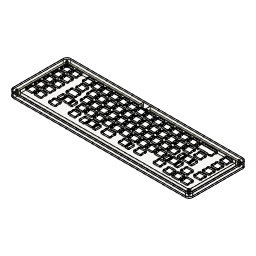
FrogdorCase (Autodesk Fusion 360 design; units mm, degrees)
Autodesk Fusion 360 part; units mm, degrees
(part 1 of 5)
sketch "plate" plane through (0, 0, 0) normal (0, 0, 1) x (1, 0, 0)
  line L0 (288.37, 77.8715) -> (287.569, 77.8715)
  line L1 (326.182, 65.8717) -> (326.981, 65.8717)
  line L2 (17.4198, 49.9223) -> (16.6192, 49.9223)
  line L3 (350.282, 78.8719) -> (350.282, 77.8715)
  line L4 (312.182, 68.9723) -> (311.381, 68.9723)
  line L5 (326.981, 65.8717) -> (326.981, 68.9723)
  line L6 (365.083, 65.8717) -> (365.083, 68.9723)
  line L7 (312.182, 77.8715) -> (311.381, 77.8715)
  line L8 (312.182, 64.8727) -> (326.182, 64.8727)
  line L9 (311.381, 74.7723) -> (312.182, 74.7723)
  line L10 (287.569, 77.8715) -> (287.569, 74.7723)
  line L11 (287.569, 74.7723) -> (288.37, 74.7723)
  line L12 (364.282, 77.8715) -> (364.282, 78.8719)
  line L13 (326.182, 74.7723) -> (326.981, 74.7723)
  line L14 (288.37, 68.9723) -> (287.569, 68.9723)
  line L15 (288.37, 74.7723) -> (288.37, 68.9723)
  line L16 (288.37, 65.8717) -> (288.37, 64.8727)
  line L17 (16.6192, 58.8215) -> (16.6192, 59.8219)
  line L18 (326.981, 74.7723) -> (326.981, 77.8715)
  line L19 (350.282, 64.8727) -> (364.282, 64.8727)
  line L20 (365.083, 68.9723) -> (364.282, 68.9723)
  line L21 (287.569, 68.9723) -> (287.569, 65.8717)
  line L22 (349.481, 65.8717) -> (350.282, 65.8717)
  line L23 (311.381, 77.8715) -> (311.381, 74.7723)
  line L24 (364.282, 74.7723) -> (365.083, 74.7723)
  line L25 (350.282, 77.8715) -> (349.481, 77.8715)
  line L26 (364.282, 68.9723) -> (364.282, 74.7723)
  line L27 (16.6192, 59.8219) -> (2.6196, 59.8219)
  line L28 (365.083, 77.8715) -> (364.282, 77.8715)
  line L29 (326.182, 77.8715) -> (326.182, 78.8719)
  line L30 (16.6192, 55.7223) -> (17.4198, 55.7223)
  line L31 (326.981, 68.9723) -> (326.182, 68.9723)
  line L32 (288.37, 64.8727) -> (302.369, 64.8727)
  line L33 (302.369, 65.8717) -> (303.17, 65.8717)
  line L34 (326.182, 64.8727) -> (326.182, 65.8717)
  line L35 (303.17, 65.8717) -> (303.17, 68.9723)
  line L36 (365.083, 74.7723) -> (365.083, 77.8715)
  line L37 (303.17, 68.9723) -> (302.369, 68.9723)
  line L38 (326.981, 77.8715) -> (326.182, 77.8715)
  line L39 (349.481, 74.7723) -> (350.282, 74.7723)
  line L40 (312.182, 65.8717) -> (312.182, 64.8727)
  line L41 (326.182, 68.9723) -> (326.182, 74.7723)
  line L42 (350.282, 68.9723) -> (349.481, 68.9723)
  line L43 (231.22, 74.7723) -> (231.22, 68.9723)
  line L44 (249.469, 65.8717) -> (250.27, 65.8717)
  line L45 (283.319, 68.9723) -> (283.319, 74.7723)
  line L46 (264.269, 77.8715) -> (264.269, 78.8719)
  line L47 (268.519, 74.7723) -> (269.32, 74.7723)
  line L48 (230.419, 77.8715) -> (230.419, 74.7723)
  line L49 (265.07, 77.8715) -> (264.269, 77.8715)
  line L50 (265.07, 65.8717) -> (265.07, 68.9723)
  line L51 (230.419, 68.9723) -> (230.419, 65.8717)
  line L52 (231.22, 78.8719) -> (231.22, 77.8715)
  line L53 (264.269, 65.8717) -> (265.07, 65.8717)
  line L54 (250.27, 78.8719) -> (250.27, 77.8715)
  line L55 (302.369, 64.8727) -> (302.369, 65.8717)
  line L56 (231.22, 77.8715) -> (230.419, 77.8715)
  line L57 (230.419, 74.7723) -> (231.22, 74.7723)
  line L58 (249.469, 74.7723) -> (250.27, 74.7723)
  line L59 (268.519, 68.9723) -> (268.519, 65.8717)
  line L60 (268.519, 65.8717) -> (269.32, 65.8717)
  line L61 (269.32, 65.8717) -> (269.32, 64.8727)
  line L62 (287.569, 65.8717) -> (288.37, 65.8717)
  line L63 (302.369, 78.8719) -> (288.37, 78.8719)
  line L64 (326.182, 78.8719) -> (312.182, 78.8719)
  line L65 (283.319, 64.8727) -> (283.319, 65.8717)
  line L66 (302.369, 77.8715) -> (302.369, 78.8719)
  line L67 (349.481, 68.9723) -> (349.481, 65.8717)
  line L68 (246.02, 65.8717) -> (246.02, 68.9723)
  line L69 (269.32, 74.7723) -> (269.32, 68.9723)
  line L70 (245.219, 65.8717) -> (246.02, 65.8717)
  line L71 (245.219, 68.9723) -> (245.219, 74.7723)
  line L72 (350.282, 65.8717) -> (350.282, 64.8727)
  line L73 (284.12, 65.8717) -> (284.12, 68.9723)
  line L74 (212.17, 78.8719) -> (212.17, 77.8715)
  line L75 (245.219, 78.8719) -> (231.22, 78.8719)
  line L76 (250.27, 77.8715) -> (249.469, 77.8715)
  line L77 (245.219, 77.8715) -> (245.219, 78.8719)
  line L78 (283.319, 65.8717) -> (284.12, 65.8717)
  line L79 (283.319, 78.8719) -> (269.32, 78.8719)
  line L80 (265.07, 74.7723) -> (265.07, 77.8715)
  line L81 (250.27, 65.8717) -> (250.27, 64.8727)
  line L82 (231.22, 65.8717) -> (231.22, 64.8727)
  line L83 (283.319, 77.8715) -> (283.319, 78.8719)
  line L84 (264.269, 74.7723) -> (265.07, 74.7723)
  line L85 (246.02, 74.7723) -> (246.02, 77.8715)
  line L86 (268.519, 77.8715) -> (268.519, 74.7723)
  line L87 (249.469, 77.8715) -> (249.469, 74.7723)
  line L88 (302.369, 74.7723) -> (303.17, 74.7723)
  line L89 (230.419, 65.8717) -> (231.22, 65.8717)
  line L90 (231.22, 64.8727) -> (245.219, 64.8727)
  line L91 (246.02, 68.9723) -> (245.219, 68.9723)
  line L92 (246.02, 77.8715) -> (245.219, 77.8715)
  line L93 (269.32, 64.8727) -> (283.319, 64.8727)
  line L94 (303.17, 74.7723) -> (303.17, 77.8715)
  line L95 (264.269, 68.9723) -> (264.269, 74.7723)
  line L96 (245.219, 64.8727) -> (245.219, 65.8717)
  line L97 (249.469, 68.9723) -> (249.469, 65.8717)
  line L98 (250.27, 64.8727) -> (264.269, 64.8727)
  line L99 (231.22, 68.9723) -> (230.419, 68.9723)
  line L100 (265.07, 68.9723) -> (264.269, 68.9723)
  line L101 (245.219, 74.7723) -> (246.02, 74.7723)
  line L102 (264.269, 78.8719) -> (250.27, 78.8719)
  line L103 (284.12, 68.9723) -> (283.319, 68.9723)
  line L104 (264.269, 64.8727) -> (264.269, 65.8717)
  line L105 (269.32, 77.8715) -> (268.519, 77.8715)
  line L106 (283.319, 74.7723) -> (284.12, 74.7723)
  line L107 (250.27, 74.7723) -> (250.27, 68.9723)
  line L108 (226.169, 78.8719) -> (212.17, 78.8719)
  line L109 (193.12, 68.9723) -> (192.319, 68.9723)
  line L110 (193.12, 78.8719) -> (193.12, 77.8715)
  line L111 (226.97, 65.8717) -> (226.97, 68.9723)
  line L112 (188.069, 64.8727) -> (188.069, 65.8717)
  line L113 (250.27, 68.9723) -> (249.469, 68.9723)
  line L114 (193.12, 65.8717) -> (193.12, 64.8727)
  line L115 (174.07, 74.7723) -> (174.07, 68.9723)
  line L116 (269.32, 68.9723) -> (268.519, 68.9723)
  line L117 (303.17, 77.8715) -> (302.369, 77.8715)
  line L118 (192.319, 77.8715) -> (192.319, 74.7723)
  line L119 (192.319, 65.8717) -> (193.12, 65.8717)
  line L120 (188.069, 65.8717) -> (188.87, 65.8717)
  line L121 (212.17, 68.9723) -> (211.369, 68.9723)
  line L122 (226.97, 74.7723) -> (226.97, 77.8715)
  line L123 (155.02, 78.8719) -> (155.02, 77.8715)
  line L124 (226.97, 68.9723) -> (226.169, 68.9723)
  line L125 (226.169, 74.7723) -> (226.97, 74.7723)
  line L126 (207.119, 68.9723) -> (207.119, 74.7723)
  line L127 (284.12, 77.8715) -> (283.319, 77.8715)
  line L128 (226.169, 77.8715) -> (226.169, 78.8719)
  line L129 (226.169, 64.8727) -> (226.169, 65.8717)
  line L130 (188.87, 65.8717) -> (188.87, 68.9723)
  line L131 (192.319, 74.7723) -> (193.12, 74.7723)
  line L132 (207.119, 74.7723) -> (207.92, 74.7723)
  line L133 (154.219, 77.8715) -> (154.219, 74.7723)
  line L134 (193.12, 77.8715) -> (192.319, 77.8715)
  line L135 (188.069, 74.7723) -> (188.87, 74.7723)
  line L136 (192.319, 68.9723) -> (192.319, 65.8717)
  line L137 (188.87, 74.7723) -> (188.87, 77.8715)
  line L138 (174.07, 68.9723) -> (173.269, 68.9723)
  line L139 (154.219, 74.7723) -> (155.02, 74.7723)
  line L140 (193.12, 74.7723) -> (193.12, 68.9723)
  line L141 (155.02, 74.7723) -> (155.02, 68.9723)
  line L142 (188.069, 77.8715) -> (188.069, 78.8719)
  line L143 (211.369, 77.8715) -> (211.369, 74.7723)
  line L144 (212.17, 74.7723) -> (212.17, 68.9723)
  line L145 (207.92, 65.8717) -> (207.92, 68.9723)
  line L146 (207.92, 68.9723) -> (207.119, 68.9723)
  line L147 (269.32, 78.8719) -> (269.32, 77.8715)
  line L148 (284.12, 74.7723) -> (284.12, 77.8715)
  line L149 (226.97, 77.8715) -> (226.169, 77.8715)
  line L150 (188.069, 68.9723) -> (188.069, 74.7723)
  line L151 (193.12, 64.8727) -> (207.119, 64.8727)
  line L152 (188.069, 78.8719) -> (174.07, 78.8719)
  line L153 (155.02, 77.8715) -> (154.219, 77.8715)
  line L154 (207.119, 77.8715) -> (207.119, 78.8719)
  line L155 (207.92, 74.7723) -> (207.92, 77.8715)
  line L156 (174.07, 64.8727) -> (188.069, 64.8727)
  line L157 (211.369, 74.7723) -> (212.17, 74.7723)
  line L158 (211.369, 65.8717) -> (212.17, 65.8717)
  line L159 (173.269, 65.8717) -> (174.07, 65.8717)
  line L160 (188.87, 77.8715) -> (188.069, 77.8715)
  line L161 (188.87, 68.9723) -> (188.069, 68.9723)
  line L162 (173.269, 74.7723) -> (174.07, 74.7723)
  line L163 (207.119, 65.8717) -> (207.92, 65.8717)
  line L164 (173.269, 68.9723) -> (173.269, 65.8717)
  line L165 (174.07, 65.8717) -> (174.07, 64.8727)
  line L166 (94.6877, 11.8222) -> (94.6877, 8.7216)
  line L167 (16.6192, 8.7216) -> (17.4198, 8.7216)
  line L168 (326.47, 23.0105) -> (326.47, 22.01)
  line L169 (325.669, 31.9098) -> (326.47, 31.9098)
  line L170 (36.4698, 17.6237) -> (36.4698, 20.7216)
  line L171 (238.362, 17.6237) -> (238.362, 11.8222)
  line L172 (16.6192, 21.722) -> (2.6196, 21.722)
  line L173 (109.488, 20.7216) -> (109.488, 21.722)
  line L174 (51.8252, 20.7216) -> (51.8252, 17.6237)
  line L175 (340.469, 36.0094) -> (326.47, 36.0094)
  line L176 (66.6253, 21.722) -> (52.626, 21.722)
  line L177 (66.6253, 20.7216) -> (66.6253, 21.722)
  line L178 (109.488, 17.6237) -> (110.287, 17.6237)
  line L179 (67.4261, 17.6237) -> (67.4261, 20.7216)
  line L180 (340.469, 22.01) -> (340.469, 23.0105)
  line L181 (341.27, 26.1097) -> (340.469, 26.1097)
  line L182 (17.4198, 20.7216) -> (16.6192, 20.7216)
  line L183 (325.669, 35.0104) -> (325.669, 31.9098)
  line L184 (325.669, 23.0105) -> (326.47, 23.0105)
  line L185 (35.669, 7.7225) -> (35.669, 8.7216)
  line L186 (293.132, 39.7715) -> (292.331, 39.7715)
  line L187 (17.4198, 17.6237) -> (17.4198, 20.7216)
  line L188 (67.4261, 8.7216) -> (67.4261, 11.8222)
  line L189 (110.287, 20.7216) -> (109.488, 20.7216)
  line L190 (326.47, 35.0104) -> (325.669, 35.0104)
  line L191 (341.27, 31.9098) -> (341.27, 35.0104)
  line L192 (21.6697, 7.7225) -> (35.669, 7.7225)
  line L193 (340.469, 26.1097) -> (340.469, 31.9098)
  line L194 (341.27, 23.0105) -> (341.27, 26.1097)
  line L195 (95.4871, 7.7225) -> (109.488, 7.7225)
  line L196 (35.669, 8.7216) -> (36.4698, 8.7216)
  line L197 (1.819, 11.8222) -> (1.819, 8.7216)
  line L198 (340.469, 35.0104) -> (340.469, 36.0094)
  line L199 (237.563, 11.8222) -> (237.563, 8.7216)
  line L200 (16.6192, 11.8222) -> (16.6192, 17.6237)
  line L201 (16.6192, 17.6237) -> (17.4198, 17.6237)
  line L202 (16.6192, 20.7216) -> (16.6192, 21.722)
  line L203 (1.819, 8.7216) -> (2.6197, 8.7216)
  line L204 (293.132, 36.6723) -> (293.132, 36.0715)
  line L205 (326.47, 22.01) -> (340.469, 22.01)
  line L206 (2.6197, 8.7216) -> (2.6197, 7.7225)
  line L207 (66.6253, 7.7225) -> (66.6253, 8.7216)
  line L208 (1.819, 17.6237) -> (2.6197, 17.6237)
  line L209 (52.626, 20.7216) -> (51.8252, 20.7216)
  line L210 (110.287, 8.7216) -> (110.287, 11.8222)
  line L211 (1.819, 20.7216) -> (1.819, 17.6237)
  line L212 (36.4698, 8.7216) -> (36.4698, 11.8222)
  line L213 (292.331, 36.6723) -> (293.132, 36.6723)
  line L214 (35.669, 17.6237) -> (36.4698, 17.6237)
  line L215 (326.47, 36.0094) -> (326.47, 35.0104)
  line L216 (17.4198, 8.7216) -> (17.4198, 11.8222)
  line L217 (36.4698, 11.8222) -> (35.669, 11.8222)
  line L218 (17.4198, 11.8222) -> (16.6192, 11.8222)
  line L219 (340.469, 31.9098) -> (341.27, 31.9098)
  line L220 (35.669, 11.8222) -> (35.669, 17.6237)
  line L221 (36.4698, 20.7216) -> (35.669, 20.7216)
  line L222 (341.27, 35.0104) -> (340.469, 35.0104)
  line L223 (21.6697, 8.7216) -> (21.6697, 7.7225)
  line L224 (340.469, 23.0105) -> (341.27, 23.0105)
  line L225 (325.669, 26.1097) -> (325.669, 23.0105)
  line L226 (35.669, 20.7216) -> (35.669, 21.722)
  line L227 (2.6197, 20.7216) -> (1.819, 20.7216)
  line L228 (2.6197, 17.6237) -> (2.6197, 11.8222)
  line L229 (293.132, 40.7719) -> (293.132, 39.7715)
  line L230 (35.669, 21.722) -> (21.6697, 21.722)
  line L231 (284.032, 36.0715) -> (284.032, 33.2727)
  line L232 (292.331, 39.7715) -> (292.331, 36.6723)
  line L233 (291.607, 36.0715) -> (291.607, 38.3016)
  line L234 (326.47, 31.9098) -> (326.47, 26.1097)
  line L235 (326.47, 26.1097) -> (325.669, 26.1097)
  line L236 (2.6197, 7.7225) -> (16.6192, 7.7225)
  line L237 (16.6192, 7.7225) -> (16.6192, 8.7216)
  line L238 (61.3502, 39.7715) -> (61.3502, 36.6737)
  line L239 (291.607, 27.0027) -> (291.607, 31.4716)
  line L240 (307.132, 27.7716) -> (307.931, 27.7716)
  line L241 (307.132, 26.7725) -> (307.132, 27.7716)
  line L242 (315.407, 39.3016) -> (315.248, 39.3016)
  line L243 (307.132, 40.7719) -> (293.132, 40.7719)
  line L244 (62.151, 39.7715) -> (61.3502, 39.7715)
  line L245 (60.6256, 36.0715) -> (60.6256, 39.3016)
  line L246 (61.3502, 36.6737) -> (62.151, 36.6737)
  line L247 (307.132, 39.7715) -> (307.132, 40.7719)
  line L248 (2.6197, 11.8222) -> (1.819, 11.8222)
  line L249 (2.6197, 21.722) -> (2.6197, 20.7216)
  line L250 (293.132, 26.7725) -> (307.132, 26.7725)
  line L251 (62.151, 36.6737) -> (62.151, 36.0715)
  line L252 (61.3502, 30.8722) -> (61.3502, 27.7716)
  line L253 (307.931, 30.8722) -> (307.132, 30.8722)
  line L254 (62.151, 40.7719) -> (62.151, 39.7715)
  line L255 (61.3502, 27.7716) -> (62.151, 27.7716)
  line L256 (60.6225, 27.0027) -> (60.6256, 27.0027)
  line L257 (307.931, 39.7715) -> (307.132, 39.7715)
  line L258 (307.132, 36.6723) -> (307.931, 36.6723)
  line L259 (62.151, 31.4716) -> (62.151, 30.8722)
  line L260 (307.931, 36.6723) -> (307.931, 39.7715)
  line L261 (60.6256, 39.3016) -> (53.8759, 39.3016)
  line L262 (60.6256, 27.0027) -> (60.6256, 31.4716)
  line L263 (316.231, 33.2727) -> (316.231, 36.0715)
  line L264 (62.151, 30.8722) -> (61.3502, 30.8722)
  line L265 (307.132, 30.8722) -> (307.132, 31.4716)
  line L266 (292.331, 27.7716) -> (293.132, 27.7716)
  line L267 (292.331, 30.8722) -> (292.331, 27.7716)
  line L268 (293.132, 27.7716) -> (293.132, 26.7725)
  line L269 (307.931, 27.7716) -> (307.931, 30.8722)
  line L270 (293.132, 31.4716) -> (293.132, 30.8722)
  line L271 (293.132, 30.8722) -> (292.331, 30.8722)
  line L272 (364.282, 36.6737) -> (365.083, 36.6737)
  line L273 (62.151, 27.7716) -> (62.151, 26.7725)
  line L274 (350.282, 39.7715) -> (349.481, 39.7715)
  line L275 (76.1503, 36.6737) -> (76.9511, 36.6737)
  line L276 (76.1503, 40.7719) -> (62.151, 40.7719)
  line L277 (350.282, 26.7725) -> (364.282, 26.7725)
  line L278 (264.557, 30.8722) -> (263.756, 30.8722)
  line L279 (350.282, 36.6737) -> (350.282, 30.8722)
  line L280 (349.481, 30.8722) -> (349.481, 27.7716)
  line L281 (278.557, 27.7716) -> (279.356, 27.7716)
  line L282 (77.676, 31.4716) -> (77.676, 27.0027)
  line L283 (350.282, 30.8722) -> (349.481, 30.8722)
  line L284 (76.9511, 39.7715) -> (76.1503, 39.7715)
  line L285 (76.9511, 36.6737) -> (76.9511, 39.7715)
  line L286 (263.756, 27.7716) -> (264.557, 27.7716)
  line L287 (76.9511, 27.7716) -> (76.9511, 30.8722)
  line L288 (349.481, 39.7715) -> (349.481, 36.6737)
  line L289 (364.282, 40.7719) -> (350.282, 40.7719)
  line L290 (264.557, 27.7716) -> (264.557, 26.7725)
  line L291 (349.481, 27.7716) -> (350.282, 27.7716)
  line L292 (76.1503, 27.7716) -> (76.9511, 27.7716)
  line L293 (365.083, 39.7715) -> (364.282, 39.7715)
  line L294 (307.132, 36.0715) -> (307.132, 36.6723)
  line L295 (263.756, 39.7715) -> (263.756, 36.6737)
  line L296 (365.083, 30.8722) -> (364.282, 30.8722)
  line L297 (264.557, 40.7719) -> (264.557, 39.7715)
  line L298 (62.151, 26.7725) -> (76.1503, 26.7725)
  line L299 (263.756, 30.8722) -> (263.756, 27.7716)
  line L300 (279.356, 27.7716) -> (279.356, 30.8722)
  line L301 (364.282, 26.7725) -> (364.282, 27.7716)
  line L302 (279.356, 30.8722) -> (278.557, 30.8722)
  line L303 (264.557, 26.7725) -> (278.557, 26.7725)
  line L304 (77.676, 38.3016) -> (77.676, 36.0715)
  line L305 (76.9511, 30.8722) -> (76.1503, 30.8722)
  line L306 (76.1503, 36.0715) -> (76.1503, 36.6737)
  line L307 (263.756, 36.6737) -> (264.557, 36.6737)
  line L308 (264.557, 36.6737) -> (264.557, 30.8722)
  line L309 (76.1503, 26.7725) -> (76.1503, 27.7716)
  line L310 (350.282, 27.7716) -> (350.282, 26.7725)
  line L311 (278.557, 26.7725) -> (278.557, 27.7716)
  line L312 (76.1503, 30.8722) -> (76.1503, 31.4716)
  line L313 (278.557, 36.6737) -> (279.356, 36.6737)
  line L314 (76.1503, 39.7715) -> (76.1503, 40.7719)
  line L315 (264.557, 39.7715) -> (263.756, 39.7715)
  line L316 (350.282, 40.7719) -> (350.282, 39.7715)
  line L317 (364.282, 30.8722) -> (364.282, 36.6737)
  line L318 (349.481, 36.6737) -> (350.282, 36.6737)
  line L319 (365.083, 36.6737) -> (365.083, 39.7715)
  line L320 (365.083, 27.7716) -> (365.083, 30.8722)
  line L321 (278.557, 30.8722) -> (278.557, 36.6737)
  line L322 (278.557, 40.7719) -> (264.557, 40.7719)
  line L323 (126.157, 39.7715) -> (126.157, 40.7719)
  line L324 (260.306, 36.6737) -> (260.306, 39.7715)
  line L325 (364.282, 39.7715) -> (364.282, 40.7719)
  line L326 (240.457, 30.8722) -> (240.457, 36.6737)
  line L327 (245.507, 26.7725) -> (259.507, 26.7725)
  line L328 (93.1072, 30.8722) -> (92.3064, 30.8722)
  line L329 (279.356, 36.6737) -> (279.356, 39.7715)
  line L330 (111.356, 36.6737) -> (112.157, 36.6737)
  line L331 (126.157, 27.7716) -> (126.956, 27.7716)
  line L332 (225.656, 27.7716) -> (226.457, 27.7716)
  line L333 (206.606, 36.6737) -> (207.407, 36.6737)
  line L334 (240.457, 36.6737) -> (241.256, 36.6737)
  line L335 (260.306, 30.8722) -> (259.507, 30.8722)
  line L336 (244.706, 27.7716) -> (245.507, 27.7716)
  line L337 (126.956, 36.6737) -> (126.956, 39.7715)
  line L338 (92.3064, 39.7715) -> (92.3064, 36.6737)
  line L339 (130.406, 36.6737) -> (131.207, 36.6737)
  line L340 (207.407, 40.7719) -> (207.407, 39.7715)
  line L341 (93.1072, 40.7719) -> (93.1072, 39.7715)
  line L342 (225.656, 39.7715) -> (225.656, 36.6737)
  line L343 (259.507, 39.7715) -> (259.507, 40.7719)
  line L344 (240.457, 40.7719) -> (226.457, 40.7719)
  line L345 (226.457, 39.7715) -> (225.656, 39.7715)
  line L346 (225.656, 36.6737) -> (226.457, 36.6737)
  line L347 (206.606, 39.7715) -> (206.606, 36.6737)
  line L348 (226.457, 36.6737) -> (226.457, 30.8722)
  line L349 (240.457, 27.7716) -> (241.256, 27.7716)
  line L350 (244.706, 30.8722) -> (244.706, 27.7716)
  line L351 (226.457, 40.7719) -> (226.457, 39.7715)
  line L352 (260.306, 27.7716) -> (260.306, 30.8722)
  line L353 (241.256, 27.7716) -> (241.256, 30.8722)
  line L354 (241.256, 39.7715) -> (240.457, 39.7715)
  line L355 (259.507, 27.7716) -> (260.306, 27.7716)
  line L356 (244.706, 39.7715) -> (244.706, 36.6737)
  line L357 (206.606, 30.8722) -> (206.606, 27.7716)
  line L358 (245.507, 27.7716) -> (245.507, 26.7725)
  line L359 (93.1072, 36.6737) -> (93.1072, 30.8722)
  line L360 (226.457, 27.7716) -> (226.457, 26.7725)
  line L361 (245.507, 40.7719) -> (245.507, 39.7715)
  line L362 (259.507, 26.7725) -> (259.507, 27.7716)
  line L363 (207.407, 30.8722) -> (206.606, 30.8722)
  line L364 (245.507, 30.8722) -> (244.706, 30.8722)
  line L365 (226.457, 26.7725) -> (240.457, 26.7725)
  line L366 (241.256, 36.6737) -> (241.256, 39.7715)
  line L367 (240.457, 26.7725) -> (240.457, 27.7716)
  line L368 (112.157, 39.7715) -> (111.356, 39.7715)
  line L369 (364.282, 27.7716) -> (365.083, 27.7716)
  line L370 (259.507, 36.6737) -> (260.306, 36.6737)
  line L371 (207.407, 39.7715) -> (206.606, 39.7715)
  line L372 (260.306, 39.7715) -> (259.507, 39.7715)
  line L373 (259.507, 30.8722) -> (259.507, 36.6737)
  line L374 (245.507, 36.6737) -> (245.507, 30.8722)
  line L375 (207.407, 36.6737) -> (207.407, 30.8722)
  line L376 (279.356, 39.7715) -> (278.557, 39.7715)
  line L377 (259.507, 40.7719) -> (245.507, 40.7719)
  line L378 (278.557, 39.7715) -> (278.557, 40.7719)
  line L379 (241.256, 30.8722) -> (240.457, 30.8722)
  line L380 (245.507, 39.7715) -> (244.706, 39.7715)
  line L381 (244.706, 36.6737) -> (245.507, 36.6737)
  line L382 (240.457, 39.7715) -> (240.457, 40.7719)
  line L383 (226.457, 30.8722) -> (225.656, 30.8722)
  line L384 (225.656, 30.8722) -> (225.656, 27.7716)
  line L385 (126.157, 36.6737) -> (126.956, 36.6737)
  line L386 (93.1072, 27.7716) -> (93.1072, 26.7725)
  line L387 (21.6697, 40.7719) -> (21.6697, 39.7715)
  line L388 (131.207, 27.7716) -> (131.207, 26.7725)
  line L389 (112.157, 27.7716) -> (112.157, 26.7725)
  line L390 (92.3064, 30.8722) -> (92.3064, 27.7716)
  line L391 (145.207, 27.7716) -> (146.006, 27.7716)
  line L392 (130.406, 30.8722) -> (130.406, 27.7716)
  line L393 (107.906, 27.7716) -> (107.906, 30.8722)
  line L394 (131.207, 40.7719) -> (131.207, 39.7715)
  line L395 (145.207, 26.7725) -> (145.207, 27.7716)
  line L396 (126.956, 30.8722) -> (126.157, 30.8722)
  line L397 (126.956, 27.7716) -> (126.956, 30.8722)
  line L398 (146.006, 30.8722) -> (145.207, 30.8722)
  line L399 (112.157, 40.7719) -> (112.157, 39.7715)
  line L400 (164.257, 39.7715) -> (164.257, 40.7719)
  line L401 (131.207, 26.7725) -> (145.207, 26.7725)
  line L402 (131.207, 30.8722) -> (130.406, 30.8722)
  line L403 (107.107, 36.6737) -> (107.906, 36.6737)
  line L404 (93.1072, 39.7715) -> (92.3064, 39.7715)
  line L405 (111.356, 27.7716) -> (112.157, 27.7716)
  line L406 (145.207, 40.7719) -> (131.207, 40.7719)
  line L407 (107.107, 27.7716) -> (107.906, 27.7716)
  line L408 (112.157, 26.7725) -> (126.157, 26.7725)
  line L409 (146.006, 27.7716) -> (146.006, 30.8722)
  line L410 (92.3064, 27.7716) -> (93.1072, 27.7716)
  line L411 (107.906, 36.6737) -> (107.906, 39.7715)
  line L412 (131.207, 39.7715) -> (130.406, 39.7715)
  line L413 (165.056, 39.7715) -> (164.257, 39.7715)
  line L414 (107.107, 30.8722) -> (107.107, 36.6737)
  line L415 (107.107, 26.7725) -> (107.107, 27.7716)
  line L416 (145.207, 39.7715) -> (145.207, 40.7719)
  line L417 (146.006, 36.6737) -> (146.006, 39.7715)
  line L418 (130.406, 39.7715) -> (130.406, 36.6737)
  line L419 (107.906, 39.7715) -> (107.107, 39.7715)
  line L420 (2.6197, 27.7716) -> (2.6197, 26.7725)
  line L421 (305.037, 55.7223) -> (305.037, 55.1215)
  line L422 (16.6192, 30.8722) -> (16.6192, 36.6737)
  line L423 (16.6192, 27.7716) -> (17.4198, 27.7716)
  line L424 (17.4198, 36.6737) -> (17.4198, 39.7715)
  line L425 (20.869, 27.7716) -> (21.6697, 27.7716)
  line L426 (36.4698, 30.8722) -> (35.669, 30.8722)
  line L427 (304.238, 55.7223) -> (305.037, 55.7223)
  line L428 (126.157, 26.7725) -> (126.157, 27.7716)
  line L429 (20.869, 39.7715) -> (20.869, 36.6737)
  line L430 (35.669, 27.7716) -> (36.4698, 27.7716)
  line L431 (130.406, 27.7716) -> (131.207, 27.7716)
  line L432 (21.6697, 26.7725) -> (35.669, 26.7725)
  line L433 (17.4198, 30.8722) -> (16.6192, 30.8722)
  line L434 (107.107, 39.7715) -> (107.107, 40.7719)
  line L435 (305.037, 59.8219) -> (305.037, 58.8215)
  line L436 (107.906, 30.8722) -> (107.107, 30.8722)
  line L437 (2.6197, 36.6737) -> (2.6197, 30.8722)
  line L438 (2.6197, 30.8722) -> (1.819, 30.8722)
  line L439 (305.037, 50.5217) -> (305.037, 49.9223)
  line L440 (305.037, 49.9223) -> (304.238, 49.9223)
  line L441 (16.6192, 39.7715) -> (16.6192, 40.7719)
  line L442 (305.037, 58.8215) -> (304.238, 58.8215)
  line L443 (35.669, 39.7715) -> (35.669, 40.7719)
  line L444 (112.157, 30.8722) -> (111.356, 30.8722)
  line L445 (1.819, 27.7716) -> (2.6197, 27.7716)
  line L446 (2.6197, 26.7725) -> (16.6192, 26.7725)
  line L447 (2.6197, 39.7715) -> (1.819, 39.7715)
  line L448 (21.6697, 36.6737) -> (21.6697, 30.8722)
  line L449 (145.207, 30.8722) -> (145.207, 36.6737)
  line L450 (36.4698, 39.7715) -> (35.669, 39.7715)
  line L451 (126.157, 40.7719) -> (112.157, 40.7719)
  line L452 (164.257, 40.7719) -> (150.257, 40.7719)
  line L453 (1.819, 36.6737) -> (2.6197, 36.6737)
  line L454 (111.356, 39.7715) -> (111.356, 36.6737)
  line L455 (17.4198, 27.7716) -> (17.4198, 30.8722)
  line L456 (303.513, 55.1215) -> (303.513, 57.3516)
  line L457 (92.3064, 36.6737) -> (93.1072, 36.6737)
  line L458 (126.956, 39.7715) -> (126.157, 39.7715)
  line L459 (131.207, 36.6737) -> (131.207, 30.8722)
  line L460 (145.207, 36.6737) -> (146.006, 36.6737)
  line L461 (111.356, 30.8722) -> (111.356, 27.7716)
  line L462 (93.1072, 26.7725) -> (107.107, 26.7725)
  line L463 (35.669, 40.7719) -> (21.6697, 40.7719)
  line L464 (20.869, 30.8722) -> (20.869, 27.7716)
  line L465 (126.157, 30.8722) -> (126.157, 36.6737)
  line L466 (17.4198, 39.7715) -> (16.6192, 39.7715)
  line L467 (107.107, 40.7719) -> (93.1072, 40.7719)
  line L468 (146.006, 39.7715) -> (145.207, 39.7715)
  line L469 (112.157, 36.6737) -> (112.157, 30.8722)
  line L470 (1.819, 30.8722) -> (1.819, 27.7716)
  line L471 (36.4698, 27.7716) -> (36.4698, 30.8722)
  line L472 (16.6192, 36.6737) -> (17.4198, 36.6737)
  line L473 (274.082, 59.8219) -> (274.082, 58.8215)
  line L474 (273.281, 55.7223) -> (274.082, 55.7223)
  line L475 (274.082, 55.7223) -> (274.082, 49.9223)
  line L476 (365.083, 46.8217) -> (365.083, 49.9223)
  line L477 (274.082, 58.8215) -> (273.281, 58.8215)
  line L478 (35.669, 36.6737) -> (36.4698, 36.6737)
  line L479 (2.6197, 40.7719) -> (2.6197, 39.7715)
  line L480 (35.669, 26.7725) -> (35.669, 27.7716)
  line L481 (364.282, 59.8219) -> (350.282, 59.8219)
  line L482 (319.837, 49.9223) -> (319.038, 49.9223)
  line L483 (349.481, 55.7223) -> (350.282, 55.7223)
  line L484 (35.669, 30.8722) -> (35.669, 36.6737)
  line L485 (350.282, 49.9223) -> (349.481, 49.9223)
  line L486 (365.083, 49.9223) -> (364.282, 49.9223)
  line L487 (364.282, 49.9223) -> (364.282, 55.7223)
  line L488 (21.6697, 27.7716) -> (21.6697, 26.7725)
  line L489 (365.083, 58.8215) -> (364.282, 58.8215)
  line L490 (304.238, 49.9223) -> (304.238, 46.8217)
  line L491 (21.6697, 30.8722) -> (20.869, 30.8722)
  line L492 (1.819, 39.7715) -> (1.819, 36.6737)
  line L493 (365.083, 55.7223) -> (365.083, 58.8215)
  line L494 (364.282, 55.7223) -> (365.083, 55.7223)
  line L495 (304.238, 46.8217) -> (305.037, 46.8217)
  line L496 (350.282, 58.8215) -> (349.481, 58.8215)
  line L497 (16.6192, 26.7725) -> (16.6192, 27.7716)
  line L498 (364.282, 58.8215) -> (364.282, 59.8219)
  line L499 (21.6697, 39.7715) -> (20.869, 39.7715)
  line L500 (319.038, 46.8217) -> (319.837, 46.8217)
  line L501 (364.282, 46.8217) -> (365.083, 46.8217)
  line L502 (349.481, 49.9223) -> (349.481, 46.8217)
  line L503 (305.037, 46.8217) -> (305.037, 45.8227)
  line L504 (319.837, 55.7223) -> (319.837, 58.8215)
  line L505 (319.038, 59.8219) -> (305.037, 59.8219)
  line L506 (350.282, 46.8217) -> (350.282, 45.8227)
  line L507 (350.282, 45.8227) -> (364.282, 45.8227)
  line L508 (319.038, 58.8215) -> (319.038, 59.8219)
  line L509 (20.869, 36.6737) -> (21.6697, 36.6737)
  line L510 (36.4698, 36.6737) -> (36.4698, 39.7715)
  line L511 (364.282, 45.8227) -> (364.282, 46.8217)
  line L512 (319.038, 55.1215) -> (319.038, 55.7223)
  line L513 (304.238, 58.8215) -> (304.238, 55.7223)
  line L514 (319.837, 58.8215) -> (319.038, 58.8215)
  line L515 (319.038, 45.8227) -> (319.038, 46.8217)
  line L516 (16.6192, 40.7719) -> (2.6196, 40.7719)
  line L517 (350.282, 59.8219) -> (350.282, 58.8215)
  line L518 (288.082, 46.8217) -> (288.881, 46.8217)
  line L519 (305.037, 45.8227) -> (319.038, 45.8227)
  line L520 (274.082, 49.9223) -> (273.281, 49.9223)
  line L521 (288.082, 45.8227) -> (288.082, 46.8217)
  line L522 (274.082, 45.8227) -> (288.082, 45.8227)
  line L523 (273.281, 58.8215) -> (273.281, 55.7223)
  line L524 (319.038, 49.9223) -> (319.038, 50.5217)
  line L525 (350.282, 55.7223) -> (350.282, 49.9223)
  line L526 (273.281, 46.8217) -> (274.082, 46.8217)
  line L527 (349.481, 58.8215) -> (349.481, 55.7223)
  line L528 (274.082, 46.8217) -> (274.082, 45.8227)
  line L529 (288.881, 49.9223) -> (288.082, 49.9223)
  line L530 (319.038, 55.7223) -> (319.837, 55.7223)
  line L531 (273.281, 49.9223) -> (273.281, 46.8217)
  line L532 (288.881, 46.8217) -> (288.881, 49.9223)
  line L533 (288.082, 49.9223) -> (288.082, 55.7223)
  line L534 (319.837, 46.8217) -> (319.837, 49.9223)
  line L535 (349.481, 46.8217) -> (350.282, 46.8217)
  line L536 (288.082, 55.7223) -> (288.881, 55.7223)
  line L537 (288.881, 55.7223) -> (288.881, 58.8215)
  line L538 (250.781, 49.9223) -> (249.982, 49.9223)
  line L539 (249.982, 49.9223) -> (249.982, 55.7223)
  line L540 (249.982, 46.8217) -> (250.781, 46.8217)
  line L541 (269.831, 46.8217) -> (269.831, 49.9223)
  line L542 (255.032, 45.8227) -> (269.032, 45.8227)
  line L543 (254.231, 46.8217) -> (255.032, 46.8217)
  line L544 (235.181, 46.8217) -> (235.982, 46.8217)
  line L545 (216.932, 46.8217) -> (216.932, 45.8227)
  line L546 (235.982, 58.8215) -> (235.181, 58.8215)
  line L547 (235.982, 49.9223) -> (235.181, 49.9223)
  line L548 (250.781, 58.8215) -> (249.982, 58.8215)
  line L549 (216.932, 45.8227) -> (230.932, 45.8227)
  line L550 (235.181, 55.7223) -> (235.982, 55.7223)
  line L551 (249.982, 58.8215) -> (249.982, 59.8219)
  line L552 (216.932, 59.8219) -> (216.932, 58.8215)
  line L553 (216.131, 58.8215) -> (216.131, 55.7223)
  line L554 (216.932, 49.9223) -> (216.131, 49.9223)
  line L555 (269.032, 59.8219) -> (255.032, 59.8219)
  line L556 (269.032, 58.8215) -> (269.032, 59.8219)
  line L557 (235.181, 49.9223) -> (235.181, 46.8217)
  line L558 (255.032, 49.9223) -> (254.231, 49.9223)
  line L559 (216.131, 49.9223) -> (216.131, 46.8217)
  line L560 (269.831, 55.7223) -> (269.831, 58.8215)
  line L561 (235.982, 55.7223) -> (235.982, 49.9223)
  line L562 (216.131, 46.8217) -> (216.932, 46.8217)
  line L563 (250.781, 55.7223) -> (250.781, 58.8215)
  line L564 (254.231, 49.9223) -> (254.231, 46.8217)
  line L565 (250.781, 46.8217) -> (250.781, 49.9223)
  line L566 (249.982, 59.8219) -> (235.982, 59.8219)
  line L567 (269.032, 49.9223) -> (269.032, 55.7223)
  line L568 (288.881, 58.8215) -> (288.082, 58.8215)
  line L569 (269.032, 55.7223) -> (269.831, 55.7223)
  line L570 (235.982, 46.8217) -> (235.982, 45.8227)
  line L571 (216.932, 55.7223) -> (216.932, 49.9223)
  line L572 (231.731, 58.8215) -> (230.932, 58.8215)
  line L573 (216.932, 58.8215) -> (216.131, 58.8215)
  line L574 (230.932, 46.8217) -> (231.731, 46.8217)
  line L575 (269.831, 58.8215) -> (269.032, 58.8215)
  line L576 (230.932, 49.9223) -> (230.932, 55.7223)
  line L577 (231.731, 49.9223) -> (230.932, 49.9223)
  line L578 (216.131, 55.7223) -> (216.932, 55.7223)
  line L579 (197.882, 59.8219) -> (197.882, 58.8215)
  line L580 (254.231, 58.8215) -> (254.231, 55.7223)
  line L581 (235.181, 58.8215) -> (235.181, 55.7223)
  line L582 (254.231, 55.7223) -> (255.032, 55.7223)
  line L583 (235.982, 59.8219) -> (235.982, 58.8215)
  line L584 (255.032, 58.8215) -> (254.231, 58.8215)
  line L585 (230.932, 55.7223) -> (231.731, 55.7223)
  line L586 (255.032, 46.8217) -> (255.032, 45.8227)
  line L587 (235.982, 45.8227) -> (249.982, 45.8227)
  line L588 (230.932, 59.8219) -> (216.932, 59.8219)
  line L589 (288.082, 58.8215) -> (288.082, 59.8219)
  line L590 (269.032, 45.8227) -> (269.032, 46.8217)
  line L591 (249.982, 45.8227) -> (249.982, 46.8217)
  line L592 (212.681, 58.8215) -> (211.882, 58.8215)
  line L593 (178.832, 59.8219) -> (178.832, 58.8215)
  line L594 (197.081, 55.7223) -> (197.882, 55.7223)
  line L595 (197.882, 45.8227) -> (211.882, 45.8227)
  line L596 (231.731, 46.8217) -> (231.731, 49.9223)
  line L597 (231.731, 55.7223) -> (231.731, 58.8215)
  line L598 (269.831, 49.9223) -> (269.032, 49.9223)
  line L599 (230.932, 58.8215) -> (230.932, 59.8219)
  line L600 (255.032, 55.7223) -> (255.032, 49.9223)
  line L601 (288.082, 59.8219) -> (274.082, 59.8219)
  line L602 (249.982, 55.7223) -> (250.781, 55.7223)
  line L603 (255.032, 59.8219) -> (255.032, 58.8215)
  line L604 (269.032, 46.8217) -> (269.831, 46.8217)
  line L605 (230.932, 45.8227) -> (230.932, 46.8217)
  line L606 (173.782, 49.9223) -> (173.782, 55.7223)
  line L607 (158.981, 58.8215) -> (158.981, 55.7223)
  line L608 (158.981, 55.7223) -> (159.782, 55.7223)
  line L609 (159.782, 49.9223) -> (158.981, 49.9223)
  line L610 (159.782, 45.8227) -> (173.782, 45.8227)
  line L611 (211.882, 55.7223) -> (212.681, 55.7223)
  line L612 (192.832, 46.8217) -> (193.631, 46.8217)
  line L613 (173.782, 46.8217) -> (174.581, 46.8217)
  line L614 (174.581, 49.9223) -> (173.782, 49.9223)
  line L615 (211.882, 45.8227) -> (211.882, 46.8217)
  line L616 (178.031, 58.8215) -> (178.031, 55.7223)
  line L617 (159.782, 59.8219) -> (159.782, 58.8215)
  line L618 (159.782, 58.8215) -> (158.981, 58.8215)
  line L619 (193.631, 46.8217) -> (193.631, 49.9223)
  line L620 (178.832, 58.8215) -> (178.031, 58.8215)
  line L621 (159.782, 55.7223) -> (159.782, 49.9223)
  line L622 (158.981, 46.8217) -> (159.782, 46.8217)
  line L623 (211.882, 59.8219) -> (197.882, 59.8219)
  line L624 (139.931, 58.8215) -> (139.931, 55.7223)
  line L625 (192.832, 58.8215) -> (192.832, 59.8219)
  line L626 (173.782, 59.8219) -> (159.782, 59.8219)
  line L627 (173.782, 58.8215) -> (173.782, 59.8219)
  line L628 (140.732, 58.8215) -> (139.931, 58.8215)
  line L629 (212.681, 55.7223) -> (212.681, 58.8215)
  line L630 (197.882, 55.7223) -> (197.882, 49.9223)
  line L631 (178.031, 46.8217) -> (178.832, 46.8217)
  line L632 (158.981, 49.9223) -> (158.981, 46.8217)
  line L633 (159.782, 46.8217) -> (159.782, 45.8227)
  line L634 (197.081, 58.8215) -> (197.081, 55.7223)
  line L635 (197.081, 49.9223) -> (197.081, 46.8217)
  line L636 (212.681, 46.8217) -> (212.681, 49.9223)
  line L637 (211.882, 46.8217) -> (212.681, 46.8217)
  line L638 (212.681, 49.9223) -> (211.882, 49.9223)
  line L639 (193.631, 55.7223) -> (193.631, 58.8215)
  line L640 (173.782, 45.8227) -> (173.782, 46.8217)
  line L641 (173.782, 55.7223) -> (174.581, 55.7223)
  line L642 (178.832, 49.9223) -> (178.031, 49.9223)
  line L643 (174.581, 55.7223) -> (174.581, 58.8215)
  line L644 (174.581, 58.8215) -> (173.782, 58.8215)
  line L645 (197.882, 46.8217) -> (197.882, 45.8227)
  line L646 (178.832, 45.8227) -> (192.832, 45.8227)
  line L647 (174.581, 46.8217) -> (174.581, 49.9223)
  line L648 (192.832, 49.9223) -> (192.832, 55.7223)
  line L649 (140.732, 59.8219) -> (140.732, 58.8215)
  line L650 (197.882, 58.8215) -> (197.081, 58.8215)
  line L651 (178.031, 49.9223) -> (178.031, 46.8217)
  line L652 (139.931, 49.9223) -> (139.931, 46.8217)
  line L653 (136.481, 55.7223) -> (136.481, 58.8215)
  line L654 (136.481, 58.8215) -> (135.682, 58.8215)
  line L655 (102.632, 46.8217) -> (102.632, 45.8227)
  line L656 (211.882, 58.8215) -> (211.882, 59.8219)
  line L657 (192.832, 55.7223) -> (193.631, 55.7223)
  line L658 (136.481, 46.8217) -> (136.481, 49.9223)
  line L659 (135.682, 58.8215) -> (135.682, 59.8219)
  line L660 (120.881, 46.8217) -> (121.682, 46.8217)
  line L661 (154.732, 55.7223) -> (155.531, 55.7223)
  line L662 (140.732, 49.9223) -> (139.931, 49.9223)
  line L663 (197.081, 46.8217) -> (197.882, 46.8217)
  line L664 (102.632, 59.8219) -> (102.632, 58.8215)
  line L665 (193.631, 49.9223) -> (192.832, 49.9223)
  line L666 (140.732, 55.7223) -> (140.732, 49.9223)
  line L667 (178.832, 55.7223) -> (178.832, 49.9223)
  line L668 (178.832, 46.8217) -> (178.832, 45.8227)
  line L669 (197.882, 49.9223) -> (197.081, 49.9223)
  line L670 (116.632, 45.8227) -> (116.632, 46.8217)
  line L671 (117.431, 49.9223) -> (116.632, 49.9223)
  line L672 (120.881, 49.9223) -> (120.881, 46.8217)
  line L673 (155.531, 55.7223) -> (155.531, 58.8215)
  line L674 (192.832, 45.8227) -> (192.832, 46.8217)
  line L675 (211.882, 49.9223) -> (211.882, 55.7223)
  line L676 (178.031, 55.7223) -> (178.832, 55.7223)
  line L677 (193.631, 58.8215) -> (192.832, 58.8215)
  line L678 (136.481, 49.9223) -> (135.682, 49.9223)
  line L679 (192.832, 59.8219) -> (178.832, 59.8219)
  line L680 (102.632, 45.8227) -> (116.632, 45.8227)
  line L681 (117.431, 58.8215) -> (116.632, 58.8215)
  line L682 (139.931, 55.7223) -> (140.732, 55.7223)
  line L683 (116.632, 55.7223) -> (117.431, 55.7223)
  line L684 (117.431, 55.7223) -> (117.431, 58.8215)
  line L685 (121.682, 46.8217) -> (121.682, 45.8227)
  line L686 (83.5822, 58.8215) -> (82.7814, 58.8215)
  line L687 (154.732, 49.9223) -> (154.732, 55.7223)
  line L688 (102.632, 49.9223) -> (101.831, 49.9223)
  line L689 (20.869, 46.8217) -> (21.6697, 46.8217)
  line L690 (155.531, 49.9223) -> (154.732, 49.9223)
  line L691 (135.682, 46.8217) -> (136.481, 46.8217)
  line L692 (101.831, 49.9223) -> (101.831, 46.8217)
  line L693 (135.682, 59.8219) -> (121.682, 59.8219)
  line L694 (101.831, 58.8215) -> (101.831, 55.7223)
  line L695 (83.5822, 49.9223) -> (82.7814, 49.9223)
  line L696 (101.831, 46.8217) -> (102.632, 46.8217)
  line L697 (102.632, 58.8215) -> (101.831, 58.8215)
  line L698 (154.732, 45.8227) -> (154.732, 46.8217)
  line L699 (101.831, 55.7223) -> (102.632, 55.7223)
  line L700 (140.732, 46.8217) -> (140.732, 45.8227)
  line L701 (155.531, 46.8217) -> (155.531, 49.9223)
  line L702 (121.682, 58.8215) -> (120.881, 58.8215)
  line L703 (121.682, 49.9223) -> (120.881, 49.9223)
  line L704 (135.682, 55.7223) -> (136.481, 55.7223)
  line L705 (72.1872, 58.8215) -> (71.3878, 58.8215)
  line L706 (35.669, 49.9223) -> (35.669, 55.7223)
  line L707 (82.7814, 58.8215) -> (82.7814, 55.7223)
  line L708 (155.531, 58.8215) -> (154.732, 58.8215)
  line L709 (135.682, 45.8227) -> (135.682, 46.8217)
  line L710 (83.5822, 59.8219) -> (83.5822, 58.8215)
  line L711 (82.7814, 46.8217) -> (83.5822, 46.8217)
  line L712 (116.632, 58.8215) -> (116.632, 59.8219)
  line L713 (116.632, 49.9223) -> (116.632, 55.7223)
  line L714 (82.7814, 55.7223) -> (83.5822, 55.7223)
  line L715 (121.682, 45.8227) -> (135.682, 45.8227)
  line L716 (120.881, 55.7223) -> (121.682, 55.7223)
  line L717 (2.6197, 58.8215) -> (1.819, 58.8215)
  line L718 (97.5815, 58.8215) -> (97.5815, 59.8219)
  line L719 (36.4698, 46.8217) -> (36.4698, 49.9223)
  line L720 (154.732, 46.8217) -> (155.531, 46.8217)
  line L721 (121.682, 55.7223) -> (121.682, 49.9223)
  line L722 (102.632, 55.7223) -> (102.632, 49.9223)
  line L723 (82.7814, 49.9223) -> (82.7814, 46.8217)
  line L724 (71.3878, 59.8219) -> (52.626, 59.8219)
  line L725 (121.682, 59.8219) -> (121.682, 58.8215)
  line L726 (117.431, 46.8217) -> (117.431, 49.9223)
  line L727 (139.931, 46.8217) -> (140.732, 46.8217)
  line L728 (36.4698, 55.7223) -> (36.4698, 58.8215)
  line L729 (97.5815, 59.8219) -> (83.5822, 59.8219)
  line L730 (98.3809, 49.9223) -> (97.5815, 49.9223)
  line L731 (97.5815, 45.8227) -> (97.5815, 46.8217)
  line L732 (120.881, 58.8215) -> (120.881, 55.7223)
  line L733 (154.732, 59.8219) -> (140.732, 59.8219)
  line L734 (116.632, 59.8219) -> (102.632, 59.8219)
  line L735 (83.5822, 46.8217) -> (83.5822, 45.8227)
  line L736 (116.632, 46.8217) -> (117.431, 46.8217)
  line L737 (83.5822, 55.7223) -> (83.5822, 49.9223)
  line L738 (97.5815, 49.9223) -> (97.5815, 55.7223)
  line L739 (72.1872, 55.7223) -> (72.1872, 58.8215)
  line L740 (140.732, 45.8227) -> (154.732, 45.8227)
  line L741 (21.6697, 55.7223) -> (21.6697, 49.9223)
  line L742 (154.732, 58.8215) -> (154.732, 59.8219)
  line L743 (135.682, 49.9223) -> (135.682, 55.7223)
  line L744 (21.6697, 45.8227) -> (35.669, 45.8227)
  line L745 (98.3809, 55.7223) -> (98.3809, 58.8215)
  line L746 (52.626, 59.8219) -> (52.626, 58.8215)
  line L747 (21.6697, 46.8217) -> (21.6697, 45.8227)
  line L748 (36.4698, 58.8215) -> (35.669, 58.8215)
  line L749 (52.626, 46.8217) -> (52.626, 45.8227)
  line L750 (52.626, 45.8227) -> (71.3878, 45.8227)
  line L751 (71.3878, 49.9223) -> (71.3878, 55.7223)
  line L752 (98.3809, 46.8217) -> (98.3809, 49.9223)
  line L753 (2.6197, 59.8219) -> (2.6197, 58.8215)
  line L754 (35.669, 46.8217) -> (36.4698, 46.8217)
  line L755 (35.669, 59.8219) -> (21.6697, 59.8219)
  line L756 (51.8252, 58.8215) -> (51.8252, 55.7223)
  line L757 (72.1872, 46.8217) -> (72.1872, 49.9223)
  line L758 (51.8252, 46.8217) -> (52.626, 46.8217)
  line L759 (35.669, 45.8227) -> (35.669, 46.8217)
  line L760 (51.8252, 55.7223) -> (52.626, 55.7223)
  line L761 (52.626, 49.9223) -> (51.8252, 49.9223)
  line L762 (20.869, 49.9223) -> (20.869, 46.8217)
  line L763 (36.4698, 49.9223) -> (35.669, 49.9223)
  line L764 (35.669, 58.8215) -> (35.669, 59.8219)
  line L765 (16.6192, 45.8227) -> (16.6192, 46.8217)
  line L766 (16.6192, 49.9223) -> (16.6192, 55.7223)
  line L767 (1.819, 49.9223) -> (1.819, 46.8217)
  line L768 (364.282, 65.8717) -> (365.083, 65.8717)
  line L769 (349.481, 77.8715) -> (349.481, 74.7723)
  line L770 (97.5815, 55.7223) -> (98.3809, 55.7223)
  line L771 (364.282, 78.8719) -> (350.282, 78.8719)
  line L772 (17.4198, 58.8215) -> (16.6192, 58.8215)
  line L773 (2.6197, 46.8217) -> (2.6197, 45.8227)
  line L774 (72.1872, 49.9223) -> (71.3878, 49.9223)
  line L775 (52.626, 58.8215) -> (51.8252, 58.8215)
  line L776 (20.869, 58.8215) -> (20.869, 55.7223)
  line L777 (1.819, 58.8215) -> (1.819, 55.7223)
  line L778 (17.4198, 46.8217) -> (17.4198, 49.9223)
  line L779 (71.3878, 45.8227) -> (71.3878, 46.8217)
  line L780 (21.6697, 49.9223) -> (20.869, 49.9223)
  line L781 (2.6197, 45.8227) -> (16.6192, 45.8227)
  line L782 (52.626, 55.7223) -> (52.626, 49.9223)
  line L783 (35.669, 55.7223) -> (36.4698, 55.7223)
  line L784 (83.5822, 45.8227) -> (97.5815, 45.8227)
  line L785 (20.869, 55.7223) -> (21.6697, 55.7223)
  line L786 (1.819, 46.8217) -> (2.6197, 46.8217)
  line L787 (71.3878, 46.8217) -> (72.1872, 46.8217)
  line L788 (21.6697, 58.8215) -> (20.869, 58.8215)
  line L789 (16.6192, 46.8217) -> (17.4198, 46.8217)
  line L790 (288.37, 78.8719) -> (288.37, 77.8715)
  line L791 (98.3809, 58.8215) -> (97.5815, 58.8215)
  line L792 (97.5815, 46.8217) -> (98.3809, 46.8217)
  line L793 (2.6197, 49.9223) -> (1.819, 49.9223)
  line L794 (302.369, 68.9723) -> (302.369, 74.7723)
  line L795 (364.282, 64.8727) -> (364.282, 65.8717)
  line L796 (17.4198, 55.7223) -> (17.4198, 58.8215)
  line L797 (312.182, 74.7723) -> (312.182, 68.9723)
  line L798 (311.381, 68.9723) -> (311.381, 65.8717)
  line L799 (311.381, 65.8717) -> (312.182, 65.8717)
  line L800 (350.282, 74.7723) -> (350.282, 68.9723)
  line L801 (51.8252, 49.9223) -> (51.8252, 46.8217)
  line L802 (21.6697, 59.8219) -> (21.6697, 58.8215)
  line L803 (71.3878, 58.8215) -> (71.3878, 59.8219)
  line L804 (71.3878, 55.7223) -> (72.1872, 55.7223)
  line L805 (1.819, 55.7223) -> (2.6197, 55.7223)
  line L806 (312.182, 78.8719) -> (312.182, 77.8715)
  line L807 (2.6197, 55.7223) -> (2.6197, 49.9223)
  line L808 (69.2947, 84.9217) -> (69.2947, 83.9227)
  line L809 (68.4939, 88.0223) -> (68.4939, 84.9217)
  line L810 (69.2947, 83.9227) -> (83.294, 83.9227)
  line L811 (68.4939, 96.9215) -> (68.4939, 93.8223)
  line L812 (106.594, 93.8223) -> (107.395, 93.8223)
  line L813 (144.694, 84.9217) -> (145.495, 84.9217)
  line L814 (179.345, 93.8223) -> (179.345, 96.9215)
  line L815 (126.445, 83.9227) -> (140.444, 83.9227)
  line L816 (178.544, 88.0223) -> (178.544, 93.8223)
  line L817 (126.445, 97.9219) -> (126.445, 96.9215)
  line L818 (159.494, 93.8223) -> (160.295, 93.8223)
  line L819 (145.495, 97.9219) -> (145.495, 96.9215)
  line L820 (163.744, 88.0223) -> (163.744, 84.9217)
  line L821 (178.544, 93.8223) -> (179.345, 93.8223)
  line L822 (126.445, 93.8223) -> (126.445, 88.0223)
  line L823 (159.494, 88.0223) -> (159.494, 93.8223)
  line L824 (126.445, 88.0223) -> (125.644, 88.0223)
  line L825 (160.295, 84.9217) -> (160.295, 88.0223)
  line L826 (159.494, 96.9215) -> (159.494, 97.9219)
  line L827 (125.644, 96.9215) -> (125.644, 93.8223)
  line L828 (197.594, 96.9215) -> (197.594, 97.9219)
  line L829 (145.495, 84.9217) -> (145.495, 83.9227)
  line L830 (159.494, 84.9217) -> (160.295, 84.9217)
  line L831 (160.295, 93.8223) -> (160.295, 96.9215)
  line L832 (126.445, 84.9217) -> (126.445, 83.9227)
  line L833 (159.494, 83.9227) -> (159.494, 84.9217)
  line L834 (88.3447, 93.8223) -> (88.3447, 88.0223)
  line L835 (103.145, 96.9215) -> (102.344, 96.9215)
  line L836 (106.594, 88.0223) -> (106.594, 84.9217)
  line L837 (125.644, 84.9217) -> (126.445, 84.9217)
  line L838 (106.594, 84.9217) -> (107.395, 84.9217)
  line L839 (140.444, 83.9227) -> (140.444, 84.9217)
  line L840 (140.444, 84.9217) -> (141.245, 84.9217)
  line L841 (145.495, 88.0223) -> (144.694, 88.0223)
  line L842 (144.694, 93.8223) -> (145.495, 93.8223)
  line L843 (122.195, 93.8223) -> (122.195, 96.9215)
  line L844 (102.344, 93.8223) -> (103.145, 93.8223)
  line L845 (69.2947, 96.9215) -> (68.4939, 96.9215)
  line L846 (178.544, 84.9217) -> (179.345, 84.9217)
  line L847 (164.545, 83.9227) -> (178.544, 83.9227)
  line L848 (125.644, 93.8223) -> (126.445, 93.8223)
  line L849 (141.245, 93.8223) -> (141.245, 96.9215)
  line L850 (141.245, 84.9217) -> (141.245, 88.0223)
  line L851 (140.444, 93.8223) -> (141.245, 93.8223)
  line L852 (140.444, 96.9215) -> (140.444, 97.9219)
  line L853 (178.544, 83.9227) -> (178.544, 84.9217)
  line L854 (145.495, 83.9227) -> (159.494, 83.9227)
  line L855 (141.245, 88.0223) -> (140.444, 88.0223)
  line L856 (163.744, 96.9215) -> (163.744, 93.8223)
  line L857 (107.395, 83.9227) -> (121.394, 83.9227)
  line L858 (163.744, 93.8223) -> (164.545, 93.8223)
  line L859 (121.394, 97.9219) -> (107.395, 97.9219)
  line L860 (145.495, 93.8223) -> (145.495, 88.0223)
  line L861 (69.2947, 93.8223) -> (69.2947, 88.0223)
  line L862 (160.295, 96.9215) -> (159.494, 96.9215)
  line L863 (125.644, 88.0223) -> (125.644, 84.9217)
  line L864 (107.395, 93.8223) -> (107.395, 88.0223)
  line L865 (144.694, 96.9215) -> (144.694, 93.8223)
  line L866 (164.545, 88.0223) -> (163.744, 88.0223)
  line L867 (126.445, 96.9215) -> (125.644, 96.9215)
  line L868 (145.495, 96.9215) -> (144.694, 96.9215)
  line L869 (69.2947, 97.9219) -> (69.2947, 96.9215)
  line L870 (160.295, 88.0223) -> (159.494, 88.0223)
  line L871 (107.395, 97.9219) -> (107.395, 96.9215)
  line L872 (179.345, 96.9215) -> (178.544, 96.9215)
  line L873 (121.394, 93.8223) -> (122.195, 93.8223)
  line L874 (141.245, 96.9215) -> (140.444, 96.9215)
  line L875 (179.345, 88.0223) -> (178.544, 88.0223)
  line L876 (178.544, 97.9219) -> (164.545, 97.9219)
  line L877 (164.545, 84.9217) -> (164.545, 83.9227)
  line L878 (178.544, 96.9215) -> (178.544, 97.9219)
  line L879 (159.494, 97.9219) -> (145.495, 97.9219)
  line L880 (179.345, 84.9217) -> (179.345, 88.0223)
  line L881 (140.444, 97.9219) -> (126.445, 97.9219)
  line L882 (140.444, 88.0223) -> (140.444, 93.8223)
  line L883 (198.395, 96.9215) -> (197.594, 96.9215)
  line L884 (164.545, 97.9219) -> (164.545, 96.9215)
  line L885 (163.744, 84.9217) -> (164.545, 84.9217)
  line L886 (164.545, 96.9215) -> (163.744, 96.9215)
  line L887 (88.3447, 97.9219) -> (88.3447, 96.9215)
  line L888 (122.195, 88.0223) -> (121.394, 88.0223)
  line L889 (16.6192, 96.9215) -> (16.6192, 97.9219)
  line L890 (64.244, 84.9217) -> (65.0448, 84.9217)
  line L891 (35.669, 83.9227) -> (35.669, 84.9217)
  line L892 (16.6192, 84.9217) -> (17.4198, 84.9217)
  line L893 (64.244, 88.0223) -> (64.244, 93.8223)
  line L894 (17.4198, 84.9217) -> (17.4198, 88.0223)
  line L895 (65.0448, 84.9217) -> (65.0448, 88.0223)
  line L896 (36.4698, 93.8223) -> (36.4698, 96.9215)
  line L897 (17.4198, 93.8223) -> (17.4198, 96.9215)
  line L898 (35.669, 97.9219) -> (21.6697, 97.9219)
  line L899 (64.244, 96.9215) -> (64.244, 97.9219)
  line L900 (1.819, 96.9215) -> (1.819, 93.8223)
  line L901 (50.2447, 84.9217) -> (50.2447, 83.9227)
  line L902 (65.0448, 96.9215) -> (64.244, 96.9215)
  line L903 (16.6192, 83.9227) -> (16.6192, 84.9217)
  line L904 (36.4698, 88.0223) -> (35.669, 88.0223)
  line L905 (36.4698, 84.9217) -> (36.4698, 88.0223)
  line L906 (36.4698, 96.9215) -> (35.669, 96.9215)
  line L907 (21.6697, 83.9227) -> (35.669, 83.9227)
  line L908 (1.819, 93.8223) -> (2.6197, 93.8223)
  line L909 (17.4198, 88.0223) -> (16.6192, 88.0223)
  line L910 (49.4439, 84.9217) -> (50.2447, 84.9217)
  line L911 (49.4439, 88.0223) -> (49.4439, 84.9217)
  line L912 (21.6697, 84.9217) -> (21.6697, 83.9227)
  line L913 (21.6697, 88.0223) -> (20.869, 88.0223)
  line L914 (2.6197, 84.9217) -> (2.6197, 83.9227)
  line L915 (1.819, 88.0223) -> (1.819, 84.9217)
  line L916 (35.669, 88.0223) -> (35.669, 93.8223)
  line L917 (64.244, 97.9219) -> (50.2447, 97.9219)
  line L918 (20.869, 88.0223) -> (20.869, 84.9217)
  line L919 (21.6697, 97.9219) -> (21.6697, 96.9215)
  line L920 (20.869, 84.9217) -> (21.6697, 84.9217)
  line L921 (65.0448, 88.0223) -> (64.244, 88.0223)
  line L922 (17.4198, 96.9215) -> (16.6192, 96.9215)
  line L923 (16.6192, 97.9219) -> (2.6196, 97.9219)
  line L924 (1.819, 84.9217) -> (2.6197, 84.9217)
  line L925 (20.869, 96.9215) -> (20.869, 93.8223)
  line L926 (16.6192, 88.0223) -> (16.6192, 93.8223)
  line L927 (50.2447, 88.0223) -> (49.4439, 88.0223)
  line L928 (21.6697, 96.9215) -> (20.869, 96.9215)
  line L929 (64.244, 93.8223) -> (65.0448, 93.8223)
  line L930 (35.669, 96.9215) -> (35.669, 97.9219)
  line L931 (50.2447, 83.9227) -> (64.244, 83.9227)
  line L932 (16.6192, 93.8223) -> (17.4198, 93.8223)
  line L933 (35.669, 84.9217) -> (36.4698, 84.9217)
  line L934 (65.0448, 93.8223) -> (65.0448, 96.9215)
  line L935 (20.869, 93.8223) -> (21.6697, 93.8223)
  line L936 (64.244, 83.9227) -> (64.244, 84.9217)
  line L937 (83.294, 97.9219) -> (69.2947, 97.9219)
  line L938 (106.594, 96.9215) -> (106.594, 93.8223)
  line L939 (103.145, 88.0223) -> (102.344, 88.0223)
  line L940 (83.294, 84.9217) -> (84.0948, 84.9217)
  line L941 (49.4439, 96.9215) -> (49.4439, 93.8223)
  line L942 (50.2447, 96.9215) -> (49.4439, 96.9215)
  line L943 (69.2947, 88.0223) -> (68.4939, 88.0223)
  line L944 (68.4939, 84.9217) -> (69.2947, 84.9217)
  line L945 (49.4439, 93.8223) -> (50.2447, 93.8223)
  line L946 (84.0948, 88.0223) -> (83.294, 88.0223)
  line L947 (121.394, 83.9227) -> (121.394, 84.9217)